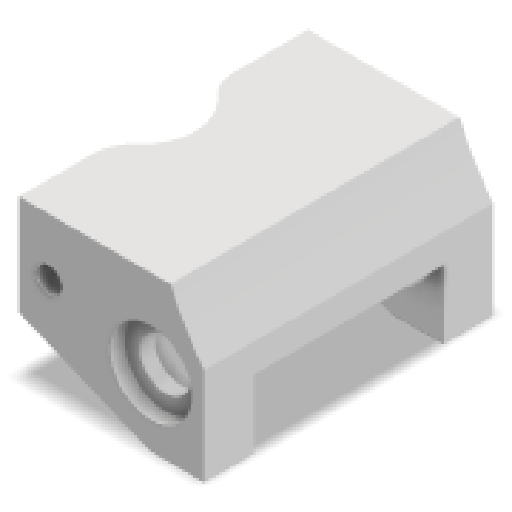
# Autodesk Inventor part: swingarmBaseV3
Saved by Autodesk Inventor 2025 (Build 290162000, 162)
## iProperties
Created: 2024-10-14
Part Number: swingarmBaseV3
Material: Generic
Document SubType Name: Modeling
Designer: derm
Density: 1 g/cm^3
Appearance: Default
Author: derm
Autodesk Inventor part; units mm, degrees
ref_plane "YZ Plane" through (0, 0, 0) normal (1, 0, 0) x (0, 1, 0)
ref_plane "XZ Plane" through (0, 0, 0) normal (0, 1, 0) x (-1, 0, 0)
ref_plane "XY Plane" through (0, 0, 0) normal (0, 0, 1) x (1, 0, 0)
sketch "Sketch1" plane through (0, 0, 0) normal (1, 0, 0) x (0, 1, 0)
  line L0 (-12.7635, 12.7635) -> (12.7635, 12.7635)
  line L1 (12.7635, 12.7635) -> (12.7635, -12.7635)
  line L2 (12.7635, -12.7635) -> (-12.7635, -12.7635)
  line L3 (-12.7635, -12.7635) -> (-12.7635, 12.7635)
  line L4 (-12.7635, 12.7635) -> (12.7635, -12.7635) construction
  line L5 (12.7635, 12.7635) -> (-12.7635, -12.7635) construction
  line L6 (19.1135, 19.1135) -> (-19.1135, 19.1135)
  line L7 (-19.1135, 19.1135) -> (-19.1135, -19.1135)
  line L8 (-19.1135, -19.1135) -> (19.1135, -19.1135)
  line L9 (19.1135, -19.1135) -> (19.1135, 19.1135)
  line L10 (12.7635, 19.1135) -> (12.7635, -19.1135)
  line L11 (-19.1135, -5.4793) -> (-46.5737, -5.4793)
  line L12 (-46.5737, -5.4793) -> (-46.5737, -19.1135)
  line L13 (-46.5737, -19.1135) -> (-19.1135, -19.1135)
  line L14 (-19.1135, -19.1135) -> (-19.1135, -5.4793)
  point P0 (0, 0)
  point P1 (12.7635, 12.7635)
  dimension "d1" = 25.527
  dimension "d2" = 6.35
  constraints: 30 end point, 6 parallel, 4 point on line, 3 perpendicular, 2 horizontal, 2 midpoint, 3 other
  measures "d1" distance of L1.end L2.end
  measures "d2" distance between parallel lines of L0 L6
extrude "Extrusion1" add sketch "Sketch1" along normal blind 50.8 contours L13 L12 L11 L7
sketch "Sketch2" plane through (0, -46.5737, -5.4793) normal (0, 0, 1) x (1, 0, 0)
  line L0 (0, 27.4602) -> (0, 0) projected
  line L1 (0, 0) -> (50.8, 0) projected
  line L2 (50.8, 27.4602) -> (50.8, 0) projected
  line L3 (0, 27.4602) -> (50.8, 27.4602) projected
  circle A0 centre (36.2123, 13.7301) radius 7
  point P0 (0, 46.5737)
  dimension "d5" = 14
  constraints: 1 centre point
  measures "d5" diameter of A0
extrude "Extrusion2" cut sketch "Sketch2" against normal through all contours A0
sketch "Sketch7" plane through (0, -46.5737, -5.4793) normal (0, 0, 1) x (1, 0, 0)
  circle A0 centre (36.2123, 13.7301) radius 7 projected
  circle A1 centre (36.2123, 13.7301) radius 11.1875
  point P0 (0, 46.5737)
  dimension "d21" = 22.375
  constraints: 1 centre point, 1 coincident
  measures "d21" diameter of A1
extrude "Extrusion7" cut sketch "Sketch7" against normal blind 4
sketch "Sketch10" plane through (0, -46.5737, -19.1135) normal (0, 0, -1) x (-1, 0, 0)
  circle A0 centre (-36.2123, 13.7301) radius 7 projected
  line L0 (0, 0) -> (0, 27.4602) projected
  line L1 (0, 27.4602) -> (-50.8, 27.4602) projected
  line L2 (-50.8, 0) -> (-50.8, 27.4602) projected
  line L3 (0, 0) -> (-50.8, 0) projected
  circle A1 centre (-36.2123, 13.7301) radius 11
  point P0 (0, 46.5737)
  constraints: 1 centre point, 1 coincident
extrude "Extrusion10" cut sketch "Sketch10" against normal blind 5.5 contours A1
sketch "Sketch11" plane through (0, -46.5737, -5.4793) normal (0, 0, 1) x (1, 0, 0)
  circle A0 centre (36.2123, 13.7301) radius 11.1875 projected
  circle A1 centre (8.2123, 21.7301) radius 2.6
  point P0 (0, 46.5737)
  dimension "d34" = 28
  dimension "d35" = 8
  dimension "d36" = 5.2
  constraints: 1 centre point
  measures "d34" horizontal distance of A0.centre A1.centre
  measures "d35" vertical distance of A0.centre A1.centre
  measures "d36" diameter of A1
extrude "Extrusion11" cut sketch "Sketch11" against normal through all contours A1
sketch "Sketch12" plane through (0, -19.1135, -5.4793) normal (0, 1, 0) x (1, 0, 0)
  line L0 (0, 13.6342) -> (0, 0) projected
  line L1 (0, 0) -> (50.8, 0) projected
  line L2 (50.8, 13.6342) -> (50.8, 0) projected
  line L3 (0, 13.6342) -> (50.8, 13.6342) projected
  point P0 (0, -5.4793)
extrude "Extrusion12" add sketch "Sketch12" along normal blind 10
sketch "Sketch13" plane through (50.8, -46.5737, -19.1135) normal (0, 0, -1) x (-1, 0, 0)
  circle A0 centre (42.5877, 21.7301) radius 2.6 projected
  circle A1 centre (14.5877, 13.7301) radius 11 projected
  line L0 (50.8, 0) -> (50.8, 37.4602) projected
  line L1 (0, 37.4602) -> (50.8, 37.4602) projected
  line L2 (0, 0) -> (0, 37.4602) projected
  line L3 (50.8, 0) -> (0, 0) projected
  line L4 (50.8, 0) -> (50.8, 37.4602) projected
  line L5 (0, 37.4602) -> (50.8, 37.4602)
  line L6 (50.8, 37.4602) -> (50.8, 28.3179)
  line L7 (50.8, 28.3179) -> (14.5877, 28.3179)
  line L8 (0, 28.3179) -> (0, 37.4602)
  arc A2 (14.5877, 28.3179) -> (0, 13.7301) centre (14.5877, 13.7301) ccw
  arc A3 (9.6596, 0) -> (19.5158, 0) centre (14.5877, 13.7301) ccw
  point P0 (50.8, 46.5737)
  constraints: 8 end point, 4 point on circle, 4 point on line, 2 centre point, 2 parallel, 2 tangent, 1 coincident, 1 horizontal, 1 perpendicular
extrude "Extrusion13" add sketch "Sketch13" along normal blind 26 contours L7 A2 L2 L1 L0
mirror "Mirror1" about plane through (25.4, -20.9786, -45.1135) normal (0, 0, -1)
fillet "Fillet5" [suppressed]
sketch "Sketch14" plane through (0, -9.1135, -5.4793) normal (0, 1, 0) x (1, 0, 0)
  line L0 (0, 0) -> (0, 79.2683) projected
  line L1 (0, 0) -> (50.8, 0) projected
  line L2 (50.8, 0) -> (50.8, 79.2683) projected
  line L3 (0, 79.2683) -> (50.8, 79.2683) projected
  circle A0 centre (-6.545, 39.6342) radius 15.197
  point P0 (0, -5.4793)
  constraints: 1 centre point
extrude "Extrusion14" cut sketch "Sketch14" against normal blind 26 contours A0 L0 | L0 A0
fillet "Fillet6" radius 10 2 edges at (0, -13.6847, -31.3981) (0, -13.6847, -58.8289)
sketch "Sketch15" plane through (50.8, -9.1135, -84.7477) normal (0, 0, -1) x (-1, 0, 0)
  line L0 (50.8, -37.4602) -> (0, -37.4602) projected
  line L1 (50.8, -37.4602) -> (50.8, 0) projected
  line L2 (50.8, 0) -> (0, 0) projected
  line L3 (0, -37.4602) -> (0, 0) projected
  circle A0 centre (42.5877, -15.7301) radius 2.6 projected
  circle A1 centre (14.5877, -23.7301) radius 11.1875 projected
  circle A2 centre (-62.5324, 30.9366) radius 78.1359
  point P0 (50.8, 9.1135)
  point P1 (0, -15.9134)
  point P2 (9.2182, 0)
  constraints: 1 centre point
extrude "Extrusion15" cut sketch "Sketch15" against normal through all contours L3 L2 A2 picked at (1.1624, -8.9232)
thicken "Thicken1" operation add thickness 1.5 both sides no extend neighbours no toward (-0.9972038, -0.0747301, 0) faces at (50.7592, -31.7535, -36.4468)
fillet "Fillet7" radius 10 1 edges at (36.2123, -18.2559, -45.1135)
sketch "Sketch16" plane through (0, -9.1135, -5.4793) normal (0, 1, 0) x (1, 0, 0)
  line L0 (41.5818, 0) -> (41.5818, 79.2683) projected
  line L1 (0, 79.2683) -> (41.5818, 79.2683) projected
  line L2 (0, 58.6382) -> (0, 79.2683) projected
  arc A0 (0, 58.6382) -> (3.4337, 51.096) centre (10, 58.6382) ccw projected
  arc A1 (3.4337, 28.1723) -> (3.4337, 51.096) centre (-6.545, 39.6342) ccw projected
  arc A2 (3.4337, 28.1723) -> (0, 20.6301) centre (10, 20.6301) ccw projected
  line L3 (0, 0) -> (0, 20.6301) projected
  line L4 (0, 0) -> (41.5818, 0) projected
  line L5 (0, 0) -> (41.5818, 0)
  line L6 (41.5818, 0) -> (41.5818, 9.8)
  line L7 (41.5818, 9.8) -> (0, 9.8)
  line L8 (0, 9.8) -> (0, 0)
  line L9 (-402.451, 35.28) -> (156.349, 35.28) projected
  line L10 (8.0732, 35.48) -> (41.5818, 35.48)
  line L11 (5.8122, 48.48) -> (41.5818, 48.48)
  line L12 (41.5818, 48.48) -> (36.5818, 48.48)
  line L13 (36.5818, 48.48) -> (36.5818, 79.2683)
  line L14 (36.5818, 79.2683) -> (41.5818, 79.2683)
  line L15 (41.5818, 79.2683) -> (41.5818, 48.48)
  line L16 (5.8122, 48.48) -> (12.8122, 48.48)
  line L17 (12.8122, 48.48) -> (12.8122, 79.2683)
  line L18 (12.8122, 79.2683) -> (5.8122, 79.2683)
  line L19 (5.8122, 79.2683) -> (5.8122, 48.48)
  point P0 (0, -5.4793)
  point P1 (0, 9.8)
  dimension "d54" = 9.8
  dimension "d55" = 0.2
  dimension "d56" = 13
  dimension "d57" = 7
  dimension "d58" = 5
  constraints: 28 end point, 8 parallel, 5 point on line, 3 horizontal, 3 perpendicular, 2 point on circle
  measures "d54" distance between parallel lines of L4 L7
  measures "d55" distance between parallel lines of L9 L10
  measures "d56" distance between parallel lines of L10 L11
  measures "d57" distance between parallel lines of L19 L17
  measures "d58" distance between parallel lines of L0 L13
extrude "Extrusion16" add sketch "Sketch16" along normal blind 25.4 contours L4 L3 L7 L0 | L10 A1 L11 L0 | L19 L1 L17 L11
sketch "Sketch17" plane through (5.8122, -9.1135, -84.7477) normal (-1, 0, 0) x (0, 0, 1)
  line L0 (0, 0) -> (30.7883, 0) projected
  line L1 (0, 0) -> (0, 25.4) projected
  line L2 (30.7883, 25.4) -> (0, 25.4) projected
  line L3 (30.7883, 0) -> (30.7883, 25.4) projected
  line L4 (30.7883, 0) -> (0, 0) projected
  line L5 (30.7883, 0) -> (30.7883, 25.4) projected
  line L6 (0, 0) -> (30.7883, 25.4)
  point P0 (84.7477, 9.1135)
  constraints: 2 end point
extrude "Extrusion17" cut sketch "Sketch17" against normal blind 25.4 contours L1 L2 L6
sketch "Sketch20" plane through (0, -46.5737, -84.7477) normal (0, 0, -1) x (-1, 0, 0)
  circle A0 centre (-8.2123, 21.7301) radius 2.6 projected
  circle A1 centre (-8.2123, 21.7301) radius 4.1
  point P0 (0, 46.5737)
  dimension "d71" = 8.2
  constraints: 1 centre point, 1 coincident
  measures "d71" diameter of A1
extrude "Extrusion20" cut sketch "Sketch20" against normal blind 8 contours A0 | A1
sketch "Sketch21" plane through (0, -46.5737, -5.4793) normal (0, 0, 1) x (1, 0, 0)
  circle A0 centre (8.2123, 21.7301) radius 2.6 projected
  circle A1 centre (8.2123, 21.7301) radius 4.1 projected
  circle A2 centre (8.2123, 21.7301) radius 3.5
  point P0 (0, 46.5737)
  dimension "d74" = 7
  constraints: 1 centre point, 1 coincident
  measures "d74" diameter of A2
extrude "Extrusion21" cut sketch "Sketch21" against normal blind 12 contours A2
sketch "Sketch22" plane through (41.5818, 16.2865, -53.9593) normal (0, 0, -1) x (-1, 0, 0)
  line L0 (444.0328, -10.536) -> (444.0328, -14.864) projected
  line L1 (444.0328, -10.536) -> (-114.7672, -10.536) projected
  line L2 (-114.7672, -14.864) -> (-114.7672, -10.536) projected
  line L3 (444.0328, -14.864) -> (-114.7672, -14.864) projected
  circle A0 centre (8.4648, -12.7) radius 2.6
  circle A1 centre (23.4097, -12.7) radius 2.6
  point P0 (41.5818, -16.2865)
  dimension "d77" = 5.2
  dimension "d78" = 5.2
  constraints: 2 centre point
  measures "d77" diameter of A0
  measures "d78" diameter of A1
extrude "Extrusion22" cut sketch "Sketch22" against normal through all contours A1 L3 L1 | L1 A1 | A1 L3 | A0 L3 L1 | L1 A0 | A0 L3
sketch "Sketch23" plane through (41.5818, 16.2865, -53.9593) normal (0, 0, -1) x (-1, 0, 0)
  circle A0 centre (23.4097, -12.7) radius 2.6 projected
  circle A1 centre (8.4648, -12.7) radius 2.6 projected
  line L0 (28.7696, -25.4) -> (28.7696, 0) projected
  line L1 (0, 0) -> (28.7696, 0) projected
  line L2 (0, -25.4) -> (0, 0) projected
  circle A2 centre (8.4648, -12.7) radius 4.5
  circle A3 centre (23.4097, -12.7) radius 4.5
  line L3 (28.7696, -25.4) -> (0, -25.4) projected
  point P0 (41.5818, -16.2865)
  dimension "d81" = 9
  dimension "d82" = 9
  constraints: 2 centre point, 2 coincident
  measures "d81" diameter of A3
  measures "d82" diameter of A2
extrude "Extrusion23" cut sketch "Sketch23" along normal mid plane 8 contours A0 | A2 | A3
ref_plane "Work Plane1" through (41.5818, -9.1135, -28.1193) normal (0, 0, -1) x (-1, 0, 0)
mirror "Mirror2" about plane through (41.5818, -9.1135, -28.1193) normal (0, 0, -1) of "Extrusion23"
fillet "Fillet9" [suppressed]
sketch "Sketch24" plane through (0, -46.5737, -84.7477) normal (0, -1, 0) x (1, 0, 0)
  line L0 (0, 79.2683) -> (0, 65.6342) projected
  line L1 (0, 65.6342) -> (50.8, 65.6342) projected
  line L2 (50.8, 79.2683) -> (50.8, 65.6342) projected
  line L3 (0, 79.2683) -> (50.8, 79.2683) projected
  line L4 (0, 0) -> (0, 13.6342) projected
  line L5 (0, 0) -> (50.8, 0) projected
  line L6 (50.8, 0) -> (50.8, 13.6342) projected
  line L7 (0, 13.6342) -> (50.8, 13.6342) projected
  point P0 (0, 84.7477)
extrude "Extrusion24" add sketch "Sketch24" along normal blind 5
sketch "Sketch25" plane through (41.5818, -9.1135, -84.7477) normal (0, 0, -1) x (-1, 0, 0)
  line L0 (-9.2182, -15.9134) -> (-9.2182, -42.4602) projected
  line L1 (41.5818, -42.4602) -> (-9.2182, -42.4602) projected
  line L2 (41.5818, -42.4602) -> (41.5818, 0) projected
  line L3 (41.5818, 0) -> (35.7696, 0) projected
  line L4 (35.7696, 0) -> (28.7696, 0) projected
  line L5 (28.7696, 0) -> (0, 0) projected
  arc A0 (-9.2182, -15.9134) -> (0, 0) centre (-71.7506, 30.9366) ccw projected
  circle A1 centre (5.3695, -23.7301) radius 11.1875 projected
  circle A2 centre (33.3695, -15.7301) radius 4.1 projected
  line L6 (5.3695, -42.4602) -> (41.5818, -27.5404)
  point P0 (41.5818, 9.1135)
  constraints: 2 end point, 2 point on line
extrude "Extrusion25" cut sketch "Sketch25" against normal through all contours L6 L2 L1
sketch "Sketch26" plane through (41.5818, -9.1135, -53.9593) normal (1, 0, 0) x (0, 0, -1)
  line L0 (30.7883, 0) -> (0, 25.4) projected
  line L1 (0, 0) -> (0, 25.4) projected
  line L2 (30.7883, 0) -> (0, 0) projected
  line L3 (-13, 0) -> (0, 0) projected
  line L4 (0, 0) -> (0, 25.4) projected
  line L5 (-13, 25.4) -> (0, 25.4) projected
  line L6 (-13, 0) -> (-13, 25.4) projected
  line L7 (-48.48, 0) -> (-38.68, 0) projected
  line L8 (-38.68, 0) -> (-38.68, 25.4) projected
  line L9 (-48.48, 25.4) -> (-38.68, 25.4) projected
  line L10 (-48.48, 0) -> (-48.48, 25.4) projected
  point P0 (-53.9593, 9.1135)
extrude "Extrusion26" cut sketch "Sketch26" against normal through all
body "Solid1"
